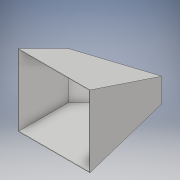
# Autodesk Inventor part: hopper
Saved by Autodesk Inventor 2019 (Build 230136000, 136)
## iProperties
Created: 2020-02-11
Part Number: hopper
Material: Generic
Document SubType Name: Modeling
Designer: ASUS
Density: 1 g/cm^3
Appearance: Default
Author: ASUS
Autodesk Inventor part; units mm, degrees
ref_plane "YZ Plane" through (0, 0, 0) normal (1, 0, 0) x (0, 1, 0)
ref_plane "XZ Plane" through (0, 0, 0) normal (0, 1, 0) x (-1, 0, 0)
ref_plane "XY Plane" through (0, 0, 0) normal (0, 0, 1) x (1, 0, 0)
sketch "Sketch1" plane through (0, 0, 0) normal (0, 1, 0) x (-1, 0, 0)
  line L0 (0, 0) -> (300, 0)
  line L1 (300, 0) -> (300, 300)
  line L2 (300, 300) -> (0, 300)
  line L3 (0, 300) -> (0, 0)
  dimension "d0" = 300
  dimension "d1" = 300
  constraints: 8 end point, 2 parallel, 1 horizontal, 1 perpendicular
  measures "d0" distance of L2.end L1.end
  measures "d1" distance of L1.end L0.end
extrude "Extrusion1" add sketch "Sketch1" along normal blind 300
chamfer "Chamfer1" distance 100 distance2 300 1 edges at (-300, 150, 0) measured on face at (-100, 100, 0)
chamfer "Chamfer2" distance 100 distance2 300 1 edges at (-100, 0, 0) measured on face at (-66.6667, 100, 0)
chamfer "Chamfer3" distance 300 distance2 100 1 edges at (-100, 300, 0) measured on face at (-166.6667, 300, 200)
chamfer "Chamfer4" distance 150 distance2 200 1 edges at (-200.0001, 150, 0) measured on face at (-266.6667, 166.6667, 199.9999)
shell "Shell1" thickness 2 removed faces 1 at (-200, 100, 300)
body "Solid1"
